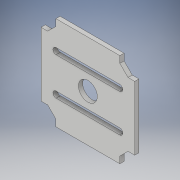
# Autodesk Inventor part: 20_Cube_insert_Sample_holder
Saved by Autodesk Inventor 2019 (Build 230136000, 136)
## iProperties
Created: 2019-08-07
Part Number: 20_Cube_insert_Sample_holder
Material: Generic
Document SubType Name: Modeling
Designer: marsikovabarbora
Density: 1 g/cm^3
Appearance: Default
Author: marsikovabarbora
Autodesk Inventor part; units mm, degrees
ref_plane "YZ Plane" through (0, 0, 0) normal (1, 0, 0) x (0, 1, 0)
ref_plane "Work Plane1" through (-29.1, -14.5, 2.4) normal (0, 0, -1) x (0, 1, 0)
ref_plane "Work Plane2" through (-13.8999, -10.5497, 2.25) normal (0, 0, -1) x (0, 1, 0)
sketch "Sketch1" plane through (0, 0, 0) normal (0, 0, 1) x (1, 0, 0)
  line L0 (-34.86, 0) -> (34.86, 0) construction
  line L1 (0, -34.86) -> (0, 34.86) construction
  line L2 (0, 0) -> (11.1575, 11.1575) construction
  line L3 (0, 0) -> (15.7791, 0) construction
  line L4 (0, 24.9) -> (16.8009, 24.9)
  line L5 (16.8009, 24.9) -> (16.8009, 21.2415)
  line L6 (16.8009, 21.2415) -> (19.0212, 19.0212)
  line L7 (24.9, 0) -> (24.9, 16.8009)
  line L8 (24.9, 16.8009) -> (21.2415, 16.8009)
  line L9 (21.2415, 16.8009) -> (19.0212, 19.0212)
  line L10 (0, -24.9) -> (16.8009, -24.9)
  line L11 (16.8009, -24.9) -> (16.8009, -21.2415)
  line L12 (16.8009, -21.2415) -> (19.0212, -19.0212)
  line L13 (24.9, 0) -> (24.9, -16.8009)
  line L14 (24.9, -16.8009) -> (21.2415, -16.8009)
  line L15 (21.2415, -16.8009) -> (19.0212, -19.0212)
  line L16 (0, 24.9) -> (-16.8009, 24.9)
  line L17 (-16.8009, 24.9) -> (-16.8009, 21.2415)
  line L18 (-16.8009, 21.2415) -> (-19.0212, 19.0212)
  line L19 (-24.9, 16.8009) -> (-21.2415, 16.8009)
  line L20 (-21.2415, 16.8009) -> (-19.0212, 19.0212)
  line L21 (0, -24.9) -> (-16.8009, -24.9)
  line L22 (-16.8009, -24.9) -> (-16.8009, -21.2415)
  line L23 (-16.8009, -21.2415) -> (-19.0212, -19.0212)
  line L24 (-21.2415, -16.8009) -> (-19.0212, -19.0212)
  line L25 (-24.9, -16.8009) -> (-21.2415, -16.8009)
  line L26 (-24.9, 0) -> (-24.9, -16.8009)
  line L27 (-24.9, 0) -> (-24.9, 16.8009)
  circle A0 centre (0, 0) radius 5
  dimension "d0" = 45
  dimension "d2" = 24.9
  dimension "d3" = 3.14
  dimension "d4" = 26.9
  dimension "d5" = 10
  constraints: 52 end point, 20 symmetric about line, 2 horizontal, 2 perpendicular, 2 point on line, 1 centre point, 1 coincident, 1 equal length
  measures "d0" angle of L3 L2
  measures "d2" distance between parallel lines of L0 L4
  measures "d3" distance of L5.end L6.end
  measures "d4" distance from line of L2.start L6
  measures "d5" diameter of A0
extrude "Extrusion1" add sketch "Sketch1" along normal up to surface (2.25 mm away)
sketch "Sketch5" plane through (0, 0, 0) normal (0, 0, -1) x (-1, 0, 0)
  circle A0 centre (-9.7, 10) radius 1.4
  circle A1 centre (-9.7, -10) radius 1.4
  circle A2 centre (13.8, 0) radius 1.4
  circle A3 centre (-10, 6.9) radius 0.75
  circle A4 centre (10, 6.9) radius 1.25
  point P0 (0, 0)
  constraints: 5 centre point, 10 other
hole "Hole1" at (9.7, -10, 0) at (9.7, 10, 0) direction (0, 0, 1) diameter 3.3 depth 12 tip angle 118
sketch "Sketch6" plane through (-16.8009, 24.9, 2.25) normal (0, 0, 1) x (1, 0, 0)
  circle A0 centre (26.5009, -34.9) radius 1.65 construction
  circle A1 centre (26.5009, -14.9) radius 1.65 construction
  circle A2 centre (16.8009, -24.9) radius 5 construction
  line L0 (33.6017, -3.6585) -> (33.6017, 0) construction
  line L1 (33.6017, 0) -> (0, 0) construction
  line L2 (0, 0) -> (0, -3.6585) construction
  line L3 (0, -3.6585) -> (-4.4406, -8.0991) construction
  line L4 (-4.4406, -8.0991) -> (-8.0991, -8.0991) construction
  line L5 (-8.0991, -8.0991) -> (-8.0991, -41.7009) construction
  line L6 (-8.0991, -41.7009) -> (-4.4406, -41.7009) construction
  line L7 (-4.4406, -41.7009) -> (0, -46.1415) construction
  line L8 (0, -46.1415) -> (0, -49.8) construction
  line L9 (0, -49.8) -> (33.6017, -49.8) construction
  line L10 (33.6017, -49.8) -> (33.6017, -46.1415) construction
  line L11 (33.6017, -46.1415) -> (38.0423, -41.7009) construction
  line L12 (38.0423, -41.7009) -> (41.7009, -41.7009) construction
  line L13 (41.7009, -41.7009) -> (41.7009, -8.0991) construction
  line L14 (41.7009, -8.0991) -> (38.0423, -8.0991) construction
  line L15 (38.0423, -8.0991) -> (33.6017, -3.6585) construction
  line L16 (33.7009, -14.9) -> (-0.0991, -14.9)
  line L17 (33.7009, -16.55) -> (-0.0991, -16.55)
  line L18 (-0.0991, -13.25) -> (33.7009, -13.25)
  arc A3 (33.7009, -16.55) -> (33.7009, -13.25) centre (33.7009, -14.9) ccw
  arc A4 (-0.0991, -13.25) -> (-0.0991, -16.55) centre (-0.0991, -14.9) ccw
  line L19 (-8.0991, -41.7009) -> (-8.0991, -8.0991) construction
  line L20 (-8.0991, -24.9) -> (41.7009, -24.9) construction
  line L21 (41.7009, -8.0991) -> (41.7009, -41.7009) construction
  circle A5 centre (26.5009, -34.9) radius 1.65 construction
  line L22 (33.7009, -34.9) -> (-0.0991, -34.9)
  line L23 (33.7009, -33.25) -> (-0.0991, -33.25)
  line L24 (-0.0991, -36.55) -> (33.7009, -36.55)
  arc A6 (33.7009, -36.55) -> (33.7009, -33.25) centre (33.7009, -34.9) ccw
  arc A7 (-0.0991, -33.25) -> (-0.0991, -36.55) centre (-0.0991, -34.9) ccw
  point P0 (16.8009, -24.9)
  point P1 (16.8009, -14.9)
  point P2 (16.8009, -34.9)
  dimension "d25" = 8
  dimension "d26" = 8
  constraints: 18 end point, 8 point on circle, 8 symmetric about line, 5 centre point, 4 tangent, 3 midpoint, 1 horizontal, 1 parallel, 3 other
  measures "d25" distance from line of L13 L16.start
  measures "d26" distance from line of L5 L16.end
extrude "Extrusion5" cut sketch "Sketch6" against normal through all
sketch "Skizze7" plane through (-16.8009, 24.9, 2.25) normal (0, 0, 1) x (1, 0, 0)
  line L0 (33.7009, -16.55) -> (-0.0991, -16.55) construction
  arc A0 (-0.0991, -13.25) -> (-0.0991, -16.55) centre (-0.0991, -14.9) ccw construction
  line L1 (-0.0991, -13.25) -> (33.7009, -13.25) construction
  arc A1 (33.7009, -16.55) -> (33.7009, -13.25) centre (33.7009, -14.9) ccw construction
  line L2 (-0.0991, -33.25) -> (33.7009, -33.25) construction
  arc A2 (33.7009, -36.55) -> (33.7009, -33.25) centre (33.7009, -34.9) ccw construction
  line L3 (33.7009, -36.55) -> (-0.0991, -36.55) construction
  arc A3 (-0.0991, -33.25) -> (-0.0991, -36.55) centre (-0.0991, -34.9) ccw construction
  circle A4 centre (16.8009, -24.9) radius 5 construction
  line L4 (33.6017, -3.6585) -> (33.6017, 0) projected
  line L5 (33.6017, 0) -> (0, 0) construction
  line L6 (0, 0) -> (0, -3.6585) projected
  line L7 (0, -3.6585) -> (-4.4406, -8.0991) projected
  line L8 (-4.4406, -8.0991) -> (-8.0991, -8.0991) projected
  line L9 (-8.0991, -8.0991) -> (-8.0991, -41.7009) construction
  line L10 (-8.0991, -41.7009) -> (-4.4406, -41.7009) projected
  line L11 (-4.4406, -41.7009) -> (0, -46.1415) projected
  line L12 (0, -46.1415) -> (0, -49.8) projected
  line L13 (0, -49.8) -> (33.6017, -49.8) construction
  line L14 (33.6017, -49.8) -> (33.6017, -46.1415) projected
  line L15 (33.6017, -46.1415) -> (38.0423, -41.7009) projected
  line L16 (38.0423, -41.7009) -> (41.7009, -41.7009) projected
  line L17 (41.7009, -41.7009) -> (41.7009, -8.0991) construction
  line L18 (41.7009, -8.0991) -> (38.0423, -8.0991) projected
  line L19 (38.0423, -8.0991) -> (33.6017, -3.6585) projected
  line L20 (-0.2, 0.2) -> (33.8017, 0.2) construction
  line L21 (33.8017, 0.2) -> (33.8017, -3.5757)
  line L22 (33.8017, -3.5757) -> (38.1252, -7.8991)
  line L23 (38.1252, -7.8991) -> (41.9009, -7.8991)
  line L24 (41.9009, -7.8991) -> (41.9009, -41.9009) construction
  line L25 (41.9009, -41.9009) -> (38.1252, -41.9009)
  line L26 (38.1252, -41.9009) -> (33.8017, -46.2243)
  line L27 (33.8017, -46.2243) -> (33.8017, -50)
  line L28 (33.8017, -50) -> (-0.2, -50) construction
  line L29 (-0.2, -50) -> (-0.2, -46.2243)
  line L30 (-0.2, -46.2243) -> (-4.5235, -41.9009)
  line L31 (-4.5235, -41.9009) -> (-8.2991, -41.9009)
  line L32 (-8.2991, -41.9009) -> (-8.2991, -7.8991) construction
  line L33 (-8.2991, -7.8991) -> (-4.5235, -7.8991)
  line L34 (-4.5235, -7.8991) -> (-0.2, -3.5757)
  line L35 (-0.2, -3.5757) -> (-0.2, 0.2)
  line L36 (33.6017, 0) -> (0, 0) projected
  line L37 (0, 0) -> (-0.2, 0)
  line L38 (-8.0991, -41.7009) -> (-8.0991, -8.0991) projected
  line L39 (-8.0991, -8.0991) -> (-8.0991, -7.8991)
  line L40 (33.6017, 0) -> (33.6017, -3.6585) projected
  line L41 (33.6017, 0) -> (33.8017, 0)
  line L42 (41.7009, -8.0991) -> (41.7009, -7.8991)
  line L43 (41.7009, -41.7009) -> (38.0423, -41.7009) projected
  line L44 (41.7009, -41.7009) -> (41.7009, -41.9009)
  line L45 (33.6017, -49.8) -> (33.8017, -49.8)
  line L46 (0, -49.8) -> (0, -46.1415) projected
  line L47 (0, -49.8) -> (-0.2, -49.8)
  line L48 (-8.0991, -41.7009) -> (-8.0991, -41.9009)
  point P0 (16.8009, -24.9)
  dimension "d29" = 0.2
  constraints: 48 end point, 11 point on line, 4 perpendicular, 1 collinear, 15 other
  measures "d29" distance between parallel lines of L5 L20
extrude "IM_offset" add sketch "Skizze7" against normal up to surface (2.25 mm away)
body "Solid1"
